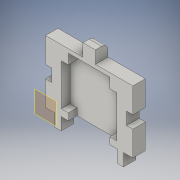
# Autodesk Inventor part: Near End Cap
Saved by Autodesk Inventor 2016 (Build 200138000, 138)
## iProperties
Created: 2016-04-25
Part Number: Near End Cap
Material: PVC-Piping
Document SubType Name: Modeling
Designer: rubenjm
Density: 1.4 g/cm^3
Appearance: Smooth - White
Author: rubenjm
Autodesk Inventor part; units mm, degrees
ref_plane "YZ Plane" through (0, 0, 0) normal (1, 0, 0) x (0, 1, 0)
ref_plane "XZ Plane" through (0, 0, 0) normal (0, 1, 0) x (-1, 0, 0)
ref_plane "XY Plane" through (0, 0, 0) normal (0, 0, 1) x (1, 0, 0)
sketch "Sketch1" plane through (0, 0, 0) normal (0, 0, 1) x (1, 0, 0)
  line L0 (0, 0) -> (9.525, 0)
  line L1 (88.9, 0) -> (88.9, 63.5)
  line L2 (88.9, 63.5) -> (0, 63.5)
  line L3 (0, 63.5) -> (0, 0)
  line L4 (79.375, 0) -> (79.375, -12.7)
  line L5 (79.375, -12.7) -> (73.025, -12.7)
  line L6 (73.025, -12.7) -> (73.025, 0)
  line L7 (44.45, 0) -> (44.45, 63.5) construction
  line L8 (16.25, 0) -> (16.25, 56.4) construction
  line L9 (16.25, 56.4) -> (72.65, 56.4) construction
  line L10 (72.65, 56.4) -> (72.65, 0) construction
  line L11 (9.525, 0) -> (9.525, -12.7)
  line L12 (9.525, -12.7) -> (15.875, -12.7)
  line L13 (15.875, -12.7) -> (15.875, 0)
  line L14 (15.875, 0) -> (73.025, 0)
  line L15 (79.375, 0) -> (88.9, 0)
  dimension "d0" = 88.9
  dimension "d1" = 63.5
  dimension "d4" = 6.35
  dimension "d5" = 12.7
  constraints: 32 end point, 4 parallel, 4 symmetric about line, 3 perpendicular, 1 collinear, 1 horizontal, 1 midpoint
  measures "d0" distance of L2.end L1.end
  measures "d1" distance of L1.end L1.start
  measures "d4" distance of L4.end L5.end
  measures "d5" distance of L4.start L4.end
ref_plane "Work Plane1" through (0, 0, 12.7) normal (0, 0, 1) x (1, 0, 0)
sketch "Sketch2" plane through (0, 0, 12.7) normal (0, 0, 1) x (1, 0, 0)
  line L0 (23.3366, 59.575) -> (23.3366, 49.3134)
  line L1 (65.5634, 51.3062) -> (65.5634, 49.3134)
  line L2 (65.5634, 59.575) -> (65.5634, 49.3134)
  line L3 (23.3366, 49.3134) -> (23.3366, 56.4)
  line L4 (65.5634, 49.3134) -> (72.65, 49.3134)
  line L5 (72.65, 49.3134) -> (72.65, 7.0866)
  line L6 (72.65, 7.0866) -> (65.5634, 7.0866)
  line L7 (23.3366, 7.0866) -> (23.3366, 0)
  line L8 (23.3366, 0) -> (65.5634, 0)
  line L9 (65.5634, 0) -> (65.5634, 7.0866)
  line L10 (23.3366, 7.0866) -> (16.25, 7.0866)
  line L11 (16.25, 7.0866) -> (16.25, 49.3134)
  line L12 (16.25, 49.3134) -> (23.3366, 49.3134)
  line L13 (44.45, 0) -> (44.45, 56.4) construction
  line L14 (28.575, 0) -> (60.325, 0) construction
  line L15 (44.45, 0) -> (44.45, 63.5) construction
  line L16 (88.9, 63.5) -> (0, 63.5) construction
  line L17 (72.65, 0) -> (16.25, 0) construction
  line L18 (16.25, 0) -> (16.25, 56.4) construction
  line L19 (72.65, 56.4) -> (72.65, 0) construction
  line L20 (23.3366, 59.575) -> (65.5634, 59.575)
  point P0 (0, 0)
  point P1 (72.65, 56.4)
  constraints: 38 end point, 5 parallel, 3 horizontal, 3 midpoint, 3 perpendicular, 3 point on line
extrude "Extrusion3" add sketch "Sketch1" along normal blind 12.7
extrude "Extrusion5" cut sketch "Sketch2" against normal blind 8.763
sketch "Sketch3" plane through (0, 0, 12.7) normal (0, 0, 1) x (1, 0, 0)
  line L0 (0, 63.5) -> (0, 0) construction
  line L1 (0, 63.5) -> (0, 0) construction
  line L2 (0, 25.4) -> (6.35, 25.4)
  line L3 (6.35, 25.4) -> (6.35, 38.1)
  line L4 (6.35, 38.1) -> (0, 38.1)
  line L5 (0, 38.1) -> (0, 25.4)
  line L6 (88.9, 63.5) -> (0, 63.5) construction
  line L7 (44.45, 63.5) -> (44.45, 0) construction
  line L8 (65.5634, 0) -> (23.3366, 0) construction
  line L9 (88.9, 25.4) -> (82.55, 25.4)
  line L10 (82.55, 25.4) -> (82.55, 38.1)
  line L11 (82.55, 38.1) -> (88.9, 38.1)
  line L12 (88.9, 38.1) -> (88.9, 25.4)
  point P0 (0, 31.75)
  point P1 (88.9, 31.75)
  dimension "d19" = 12.7
  constraints: 20 end point, 5 symmetric about line, 3 midpoint, 1 horizontal, 1 parallel, 1 perpendicular, 1 vertical
  measures "d19" distance of L3.end L2.end
extrude "Extrusion6" cut sketch "Sketch3" against normal through all
sketch "Sketch4" plane through (0, 0, 12.7) normal (0, 0, 1) x (1, 0, 0)
  line L0 (88.9, 63.5) -> (0, 63.5) construction
  line L1 (44.45, 63.5) -> (44.45, 69.85) construction
  line L2 (44.45, 63.5) -> (50.8, 63.5) construction
  line L3 (38.1, 63.5) -> (50.8, 63.5)
  line L4 (50.8, 63.5) -> (50.8, 76.2)
  line L5 (50.8, 76.2) -> (38.1, 76.2)
  line L6 (38.1, 76.2) -> (38.1, 63.5)
  line L7 (38.1, 63.5) -> (50.8, 76.2) construction
  line L8 (50.8, 63.5) -> (38.1, 76.2) construction
  point P0 (0, 0)
  dimension "d22" = 6.35
  dimension "d23" = 90
  dimension "d24" = 12.7
  dimension "d25" = 12.7
  constraints: 16 end point, 3 midpoint, 2 horizontal, 2 parallel, 2 perpendicular, 1 vertical
  measures "d22" distance of L1.start L1.end
  measures "d23" angle of L2 L1
  measures "d24" distance of L5.end L4.end
  measures "d25" distance of L4.end L3.end
extrude "Extrusion7" add sketch "Sketch4" against normal blind 12.7
fillet "Fillet1" radius 6.35 1 edges at (44.45, 76.2, 0)
body "Solid1"
